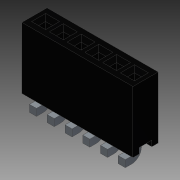
# Autodesk Inventor part: FemalConnector
Saved by Autodesk Inventor 2013 (Build 170138000, 138)
## iProperties
Created: 2015-07-05
Part Number: FemalConnector
Material: Ogólny
Document SubType Name: Modeling
Designer: terg
Density: 1 g/cm^3
Author: terg
Autodesk Inventor part; units mm, degrees
ref_plane "YZ Plane" through (0, 0, 0) normal (1, 0, 0) x (0, 1, 0)
ref_plane "XZ Plane" through (0, 0, 0) normal (0, 1, 0) x (-1, 0, 0)
sketch "Szkic1" plane through (0, 0, 0) normal (0, 0, 1) x (1, 0, 0)
  line L0 (0, 0) -> (7.94, 0)
  line L1 (7.94, 0) -> (7.94, 1.8)
  line L2 (7.94, 1.8) -> (0, 1.8)
  line L3 (0, 1.8) -> (0, 0)
  dimension "d0" = 7.94
  dimension "d1" = 1.8
  constraints: 8 end point, 2 parallel, 1 horizontal, 1 perpendicular
  measures "d0" distance of L2.end L1.end
  measures "d1" distance of L1.end L0.end
extrude "Wyciągnięcie proste1" add sketch "Szkic1" against normal blind 4.4
sketch "Szkic2" plane through (0, 0, -4.4) normal (0, 0, -1) x (-1, 0, 0)
  line L0 (-7.94, 0) -> (0, 0) projected
  line L1 (0, 0) -> (0, 1.8) projected
  line L2 (0, 1.8) -> (-7.94, 1.8) projected
  line L3 (-7.94, 1.8) -> (-7.94, 0) projected
  line L4 (-7.94, 1.8) -> (0, 1.8)
  line L5 (0, 1.8) -> (0, 1.35)
  line L6 (0, 1.35) -> (-7.94, 1.35)
  line L7 (-7.94, 1.35) -> (-7.94, 1.8)
  line L8 (-7.94, 0.45) -> (0, 0.45)
  line L9 (0, 0.45) -> (0, 0)
  line L10 (0, 0) -> (-7.94, 0)
  line L11 (-7.94, 0) -> (-7.94, 0.45)
  line L12 (-7.94, 1.35) -> (0, 1.35)
  line L13 (0, 1.35) -> (0, 0.45)
  line L14 (0, 0.45) -> (-7.94, 0.45)
  line L15 (-7.94, 0.45) -> (-7.94, 1.35)
  dimension "d4" = 0.45
  dimension "d6" = 0.45
  dimension "d7" = 1.8
  constraints: 24 end point, 6 parallel, 3 horizontal, 3 perpendicular, 2 point on line
  measures "d4" distance between parallel lines of L10 L8
  measures "d6" distance between parallel lines of L2 L6
  measures "d7" distance between parallel lines of L0 L2
extrude "Wyciągnięcie proste2" cut sketch "Szkic2" against normal blind 0.4 contours L3 L6 L1 L8
sketch "Szkic3" plane through (0, 0, 0) normal (0, 0, 1) x (1, 0, 0)
  line L0 (0, 0) -> (7.94, 0) projected
  line L1 (7.94, 1.8) -> (0, 1.8) projected
  line L2 (0, 1.8) -> (0, 0) projected
  line L3 (0.545, 1.15) -> (1.045, 1.15)
  line L4 (1.045, 1.15) -> (1.045, 0.65)
  line L5 (1.045, 0.65) -> (0.545, 0.65)
  line L6 (0.545, 0.65) -> (0.545, 1.15)
  line L7 (1.815, 1.15) -> (2.315, 1.15)
  line L8 (2.315, 1.15) -> (2.315, 0.65)
  line L9 (2.315, 0.65) -> (1.815, 0.65)
  line L10 (1.815, 0.65) -> (1.815, 1.15)
  line L11 (3.085, 1.15) -> (3.585, 1.15)
  line L12 (3.585, 1.15) -> (3.585, 0.65)
  line L13 (3.585, 0.65) -> (3.085, 0.65)
  line L14 (3.085, 0.65) -> (3.085, 1.15)
  line L15 (4.355, 1.15) -> (4.855, 1.15)
  line L16 (4.855, 1.15) -> (4.855, 0.65)
  line L17 (4.855, 0.65) -> (4.355, 0.65)
  line L18 (4.355, 0.65) -> (4.355, 1.15)
  line L19 (5.625, 1.15) -> (6.125, 1.15)
  line L20 (6.125, 1.15) -> (6.125, 0.65)
  line L21 (6.125, 0.65) -> (5.625, 0.65)
  line L22 (5.625, 0.65) -> (5.625, 1.15)
  line L23 (6.895, 1.15) -> (7.395, 1.15)
  line L24 (7.395, 1.15) -> (7.395, 0.65)
  line L25 (7.395, 0.65) -> (6.895, 0.65)
  line L26 (6.895, 0.65) -> (6.895, 1.15)
  dimension "d10" = 0.5
  dimension "d12" = 0.5
  dimension "d13" = 0.65
  dimension "d14" = 0.65
  dimension "d15" = 0.545
  dimension "d18" = 1.27
  constraints: 48 end point, 2 horizontal, 2 parallel, 1 perpendicular, 40 other
  measures "d10" distance of L3.start L3.end
  measures "d12" distance of L5.end L3.start
  measures "d13" distance between parallel lines of L1 L3
  measures "d14" distance between parallel lines of L0 L5
  measures "d15" distance between parallel lines of L2 L6
  measures "d18" distance of L3.start L7.start
extrude "Wyciągnięcie proste3" cut sketch "Szkic3" against normal blind 4
chamfer "Faza1" distance 0.25 angle 45 24 edges at (0.795, 1.15, 0) (1.045, 0.9, 0) (0.795, 0.65, 0) (0.545, 0.9, 0) (1.815, 0.9, 0) (2.065, 1.15, 0) (2.315, 0.9, 0) (2.065, 0.65, 0) (3.335, 0.65, 0) (3.085, 0.9, 0) (3.335, 1.15, 0) (3.585, 0.9, 0) (4.355, 0.9, 0) (4.605, 1.15, 0) (4.855, 0.9, 0) (4.605, 0.65, 0) (5.625, 0.9, 0) (5.875, 1.15, 0) (6.125, 0.9, 0) (5.875, 0.65, 0) (6.895, 0.9, 0) (7.145, 1.15, 0) (7.395, 0.9, 0) (7.145, 0.65, 0)
sketch "Szkic4" plane through (0, 0, -4) normal (0, 0, -1) x (-1, 0, 0)
  line L0 (-7.94, 0.45) -> (-7.94, 1.35) projected
  line L1 (-7.395, 1.15) -> (-6.895, 1.15)
  line L2 (-6.895, 1.15) -> (-6.895, 0.65)
  line L3 (-6.895, 0.65) -> (-7.395, 0.65)
  line L4 (-7.395, 0.65) -> (-7.395, 1.15)
  line L5 (-6.125, 1.15) -> (-5.625, 1.15)
  line L6 (-5.625, 1.15) -> (-5.625, 0.65)
  line L7 (-5.625, 0.65) -> (-6.125, 0.65)
  line L8 (-6.125, 0.65) -> (-6.125, 1.15)
  line L9 (-4.855, 1.15) -> (-4.355, 1.15)
  line L10 (-4.355, 1.15) -> (-4.355, 0.65)
  line L11 (-4.355, 0.65) -> (-4.855, 0.65)
  line L12 (-4.855, 0.65) -> (-4.855, 1.15)
  line L13 (-3.585, 1.15) -> (-3.085, 1.15)
  line L14 (-3.085, 1.15) -> (-3.085, 0.65)
  line L15 (-3.085, 0.65) -> (-3.585, 0.65)
  line L16 (-3.585, 0.65) -> (-3.585, 1.15)
  line L17 (-2.315, 1.15) -> (-1.815, 1.15)
  line L18 (-1.815, 1.15) -> (-1.815, 0.65)
  line L19 (-1.815, 0.65) -> (-2.315, 0.65)
  line L20 (-2.315, 0.65) -> (-2.315, 1.15)
  line L21 (-1.045, 1.15) -> (-0.545, 1.15)
  line L22 (-0.545, 1.15) -> (-0.545, 0.65)
  line L23 (-0.545, 0.65) -> (-1.045, 0.65)
  line L24 (-1.045, 0.65) -> (-1.045, 1.15)
  point P0 (0, 0)
  constraints: 48 end point, 12 parallel, 6 horizontal, 6 perpendicular
sketch "Szkic5" plane through (0, 0, 0) normal (0, -1, 0) x (1, 0, 0)
  line L0 (0, 0) -> (7.94, 0) projected
  line L1 (0, 0) -> (0, -4.4) projected
  line L2 (7.94, -4.4) -> (0, -4.4) projected
  line L3 (7.94, 0) -> (7.94, -4.4) projected
  line L4 (7.345, -4.9) -> (6.945, -4.9)
  line L5 (6.945, -4.9) -> (6.945, -5.3)
  line L6 (6.945, -5.3) -> (7.345, -5.3)
  line L7 (7.345, -5.3) -> (7.345, -4.9)
  line L8 (6.075, -4.9) -> (5.675, -4.9)
  line L9 (5.675, -4.9) -> (5.675, -5.3)
  line L10 (5.675, -5.3) -> (6.075, -5.3)
  line L11 (6.075, -5.3) -> (6.075, -4.9)
  line L12 (4.805, -4.9) -> (4.405, -4.9)
  line L13 (4.405, -4.9) -> (4.405, -5.3)
  line L14 (4.405, -5.3) -> (4.805, -5.3)
  line L15 (4.805, -5.3) -> (4.805, -4.9)
  line L16 (3.535, -4.9) -> (3.135, -4.9)
  line L17 (3.135, -4.9) -> (3.135, -5.3)
  line L18 (3.135, -5.3) -> (3.535, -5.3)
  line L19 (3.535, -5.3) -> (3.535, -4.9)
  line L20 (2.265, -4.9) -> (1.865, -4.9)
  line L21 (1.865, -4.9) -> (1.865, -5.3)
  line L22 (1.865, -5.3) -> (2.265, -5.3)
  line L23 (2.265, -5.3) -> (2.265, -4.9)
  line L24 (0.995, -4.9) -> (0.595, -4.9)
  line L25 (0.595, -4.9) -> (0.595, -5.3)
  line L26 (0.595, -5.3) -> (0.995, -5.3)
  line L27 (0.995, -5.3) -> (0.995, -4.9)
  dimension "d28" = 0.4
  dimension "d29" = 0.4
  dimension "d32" = 1.27
  dimension "d37" = 0.595
  dimension "d38" = 0.595
  dimension "d39" = 0.5
  constraints: 48 end point, 2 horizontal, 2 parallel, 1 perpendicular, 40 other
  measures "d28" distance of L6.end L5.end
  measures "d29" distance of L5.end L4.end
  measures "d32" distance of L4.start L8.start
  measures "d37" distance between parallel lines of L3 L7
  measures "d38" distance between parallel lines of L1 L25
  measures "d39" distance between parallel lines of L2 L8
ref_plane "Płaszczyzna konstrukcyjna1" through (7.145, 0.65, -4) normal (1, 0, 0) x (0, 0, -1)
sketch "Szkic6" plane through (7.145, 0.65, -4) normal (1, 0, 0) x (0, 0, -1)
  line L0 (1.3, -0.65) -> (0.9, -0.65) projected
  line L1 (0, -0.2) -> (0, 0.7) projected
  line L2 (-3.75, 0.5) -> (0, 0.5) projected
  line L3 (-3.75, 0) -> (0, 0) projected
  line L4 (0, 0.5) -> (0.6, 0.5)
  line L5 (1.3, -0.65) -> (1.3, -0.25)
  line L6 (1.3, -0.65) -> (1.7, -0.65) construction
  arc A0 (1.3, -0.25) -> (0.6, 0.5) centre (0.6, -0.2017) ccw
  point P0 (-4, -0.65)
  dimension "d40" = 0.6
  dimension "d41" = 0.4
  dimension "d42" = 90
  constraints: 6 end point, 2 perpendicular, 2 point on circle, 1 centre point, 1 horizontal, 1 parallel, 1 tangent
  measures "d40" distance of L2.end L4.end
  measures "d41" distance of L0.start L5.end
  measures "d42" angle of L6 L5
sweep "Przeciągnięcie1" add profiles "Szkic4" path "Szkic6" path curves L4 A0 L5 contours L1 L2 L3 L4
pattern_linear "Szyk prostokątny1" count 6 spacing 1.27 along (-1, 0, 0) of "Przeciągnięcie1"
equation "\"d4\" = 0.25 * d7"
equation "\"d6\" = 0.25 * d7"
equation "\"d13\" = d14"
equation "\"d37\" = d38"
